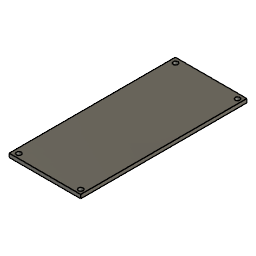
raspberry_pi_pico_mounting_board_v1 (Autodesk Fusion 360 design; units mm, degrees)
Autodesk Fusion 360 part; units mm, degrees
sketch "Sketch1" plane through (0, 0, 0) normal (0, 0, 1) x (1, 0, 0)
  line L0 (0, 0) -> (30.2, 0)
  line L1 (30.2, 0) -> (30.2, 70.15)
  line L2 (30.2, 70.15) -> (0, 70.15)
  line L3 (0, 70.15) -> (0, 0)
  dimension "d1" = 30.2
  dimension "d2" = 70.15
  constraint horizontal L0
  constraint vertical L1
  constraint horizontal L2
  constraint vertical L3
  constraint coincident L0.start L3.end
  measures "d1" distance of L0.start L0.end
  measures "d2" distance of L0.start L2.end
extrude "Extrude1" add sketch "Sketch1" along normal blind 1.6
sketch "Sketch3" plane through (0, 0, 1.6) normal (0, 0, 1) x (-1, 0, 0)
  line L0 (0, -70.15) -> (0, 0)
  line L1 (0, 0) -> (-30.2, 0)
  line L2 (-30.2, 0) -> (-30.2, -70.15)
  line L3 (-30.2, -70.15) -> (0, -70.15)
  circle A0 centre (-2.2, -68.05) radius 1
  circle A1 centre (-28.35, -68.05) radius 1
  circle A2 centre (-2.2, -1.9) radius 1
  circle A3 centre (-28.35, -1.9) radius 1
  dimension "d7" = 2
  dimension "d12" = -26.15
  dimension "d13" = 66.15
  measures "d7" diameter of A0
extrude "Extrude2" cut sketch "Sketch3" against normal blind 1.6 contours A0 | A1 | A2 | A3
